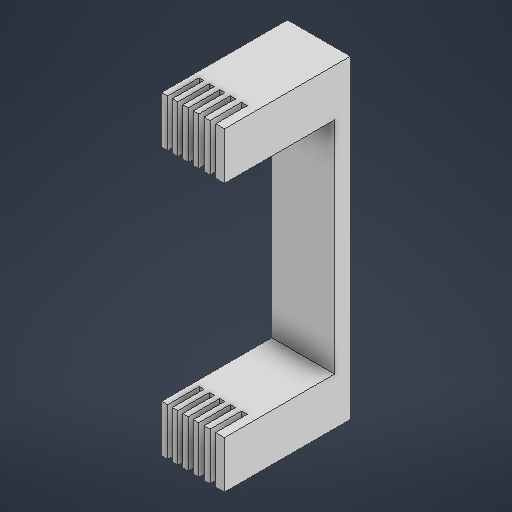
# Autodesk Inventor part: 5 nerve model
Saved by Autodesk Inventor 2026.1 (Build 301233020, 233B)
## iProperties
Created: 2025-10-27
Part Number: 5 nerve model
Material: Generisch
Document SubType Name: Modeling
Designer: sarae
Density: 1 g/cm^3
Appearance: Vorgabe
Author: sarae
Autodesk Inventor part; units mm, degrees
ref_plane "YZ Plane" through (0, 0, 0) normal (1, 0, 0) x (0, 1, 0)
ref_plane "XZ Plane" through (0, 0, 0) normal (0, 1, 0) x (-1, 0, 0)
ref_plane "XY Plane" through (0, 0, 0) normal (0, 0, 1) x (1, 0, 0)
sketch "Skizze1" plane through (0, 0, 0) normal (0, 1, 0) x (-1, 0, 0)
  line L0 (2.0157, 10.9685) -> (-1.9843, 10.9685)
  line L1 (-1.9843, 10.9685) -> (-1.9843, -9.0315)
  line L2 (-1.9843, -9.0315) -> (2.0157, -9.0315)
  line L3 (2.0157, -9.0315) -> (2.0157, 10.9685)
  point P0 (0, 0)
  dimension "d0" = 4
  dimension "d1" = 20
  constraints: 8 end point, 2 parallel, 1 horizontal, 1 perpendicular
  measures "d0" distance of L2.end L1.end
  measures "d1" distance of L1.end L0.end
extrude "Extrusion1" add sketch "Skizze1" along normal blind 1
sketch "Skizze2" plane through (0, 0, 0) normal (0, -1, 0) x (1, 0, 0)
  line L0 (-2.0157, -9.0315) -> (-2.0157, 10.9685) projected
  line L1 (-2.0157, 10.9685) -> (1.9843, 10.9685)
  line L2 (1.9843, 10.9685) -> (1.9843, 7.9685)
  line L3 (1.9843, 7.9685) -> (-2.0157, 7.9685)
  line L4 (-2.0157, 7.9685) -> (-2.0157, 10.9685)
  line L5 (-2.0157, -9.0315) -> (1.9843, -9.0315)
  line L6 (1.9843, -9.0315) -> (1.9843, -6.0315)
  line L7 (1.9843, -6.0315) -> (-2.0157, -6.0315)
  line L8 (-2.0157, -6.0315) -> (-2.0157, -9.0315)
  point P0 (0, 0)
  dimension "d4" = 4
  dimension "d5" = 3
  dimension "d6" = 4
  dimension "d7" = 3
  constraints: 16 end point, 4 parallel, 2 horizontal, 2 perpendicular
  measures "d4" distance of L2.end L3.end
  measures "d5" distance of L1.end L2.end
  measures "d6" distance of L7.end L6.end
  measures "d7" distance of L6.end L5.end
extrude "Extrusion2" add sketch "Skizze2" along normal blind 5
sketch "Skizze3" plane through (0, -5, 0) normal (0, -1, 0) x (1, 0, 0)
  line L0 (1.9843, -9.0315) -> (-2.0157, -9.0315) projected
  line L1 (-2.0157, -6.0315) -> (-1.6314, -6.0315)
  line L2 (-1.6314, -6.0315) -> (-1.6314, -9.0315)
  line L3 (-1.6314, -9.0315) -> (-2.0157, -9.0315)
  line L4 (-2.0157, -9.0315) -> (-2.0157, -6.0315)
  line L5 (1.4255, -6.0315) -> (1.9843, -6.0315)
  line L6 (1.9843, -6.0315) -> (1.9843, -9.0315)
  line L7 (1.9843, -9.0315) -> (1.4255, -9.0315)
  line L8 (1.4255, -9.0315) -> (1.4255, -6.0315)
  line L9 (-1.3305, -6.0315) -> (-0.982, -6.0315)
  line L10 (-0.982, -6.0315) -> (-0.982, -9.0315)
  line L11 (-0.982, -9.0315) -> (-1.3305, -9.0315)
  line L12 (-1.3305, -9.0315) -> (-1.3305, -6.0315)
  line L13 (0, -6.0315) -> (0.3485, -6.0315)
  line L14 (0.3485, -6.0315) -> (0.3485, -9.0315)
  line L15 (0.3485, -9.0315) -> (0, -9.0315)
  line L16 (0, -9.0315) -> (0, -6.0315)
  line L17 (-0.6651, -6.0315) -> (-0.3168, -6.0315)
  line L18 (-0.3168, -6.0315) -> (-0.3168, -9.0315)
  line L19 (-0.3168, -9.0315) -> (-0.6651, -9.0315)
  line L20 (-0.6651, -9.0315) -> (-0.6651, -6.0315)
  line L21 (1.9843, -6.0315) -> (-2.0157, -6.0315) projected
  line L22 (0.6811, -6.0315) -> (1.0612, -6.0315)
  line L23 (1.0612, -6.0315) -> (1.0612, -9.0315)
  line L24 (1.0612, -9.0315) -> (0.6811, -9.0315)
  line L25 (0.6811, -9.0315) -> (0.6811, -6.0315)
  line L26 (-0.6651, 10.9685) -> (-0.3168, 10.9685)
  line L27 (0, 10.9685) -> (0.3485, 10.9685)
  line L28 (-1.6314, 10.9685) -> (-1.6314, 7.9685)
  line L29 (-2.0157, 7.9685) -> (-2.0157, 10.9685)
  line L30 (-1.6314, 7.9685) -> (-2.0157, 7.9685)
  line L31 (0.6811, 10.9685) -> (1.0612, 10.9685)
  line L32 (-0.6651, 7.9685) -> (-0.6651, 10.9685)
  line L33 (-0.3168, 10.9685) -> (-0.3168, 7.9685)
  line L34 (-0.3168, 7.9685) -> (-0.6651, 7.9685)
  line L35 (0, 7.9685) -> (0, 10.9685)
  line L36 (0.3485, 10.9685) -> (0.3485, 7.9685)
  line L37 (0.6811, 7.9685) -> (0.6811, 10.9685)
  line L38 (1.0612, 10.9685) -> (1.0612, 7.9685)
  line L39 (1.0612, 7.9685) -> (0.6811, 7.9685)
  line L40 (1.4255, 7.9685) -> (1.4255, 10.9685)
  line L41 (1.9843, 10.9685) -> (1.9843, 7.9685)
  line L42 (-2.0157, 10.9685) -> (-1.6314, 10.9685)
  line L43 (1.4255, 10.9685) -> (1.9843, 10.9685)
  line L44 (0.3485, 7.9685) -> (0, 7.9685)
  line L45 (1.9843, 7.9685) -> (1.4255, 7.9685)
  line L46 (-0.982, 7.9685) -> (-1.3305, 7.9685)
  line L47 (-1.3305, 10.9685) -> (-0.982, 10.9685)
  line L48 (-1.3305, 7.9685) -> (-1.3305, 10.9685)
  line L49 (-0.982, 10.9685) -> (-0.982, 7.9685)
  point P0 (0, 0)
  point P1 (0, -9.0315)
  dimension "d12" = 17
  constraints: 96 end point, 14 point on line, 12 parallel, 6 horizontal, 6 perpendicular, 1 collinear, 1 vertical, 50 other
  measures "d12" distance of L1.start L29.end
extrude "Extrusion3" add sketch "Skizze3" along normal blind 2 contours L0 L8 L5 L6 | L0 L25 L21 L23 | L0 L16 L13 L14 | L0 L20 L17 L18 | L0 L12 L9 L10 | L0 L4 L1 L2 | L26 L33 L34 L32 | L27 L36 L44 L35 | L28 L30 L29 L42 | L31 L38 L39 L37 | L40 L43 L41 L45 | L46 L48 L47 L49
